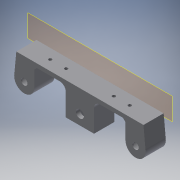
# Autodesk Inventor part: Bed Slide
Saved by Autodesk Inventor 2016 (Build 200138000, 138)
## iProperties
Created: 2016-04-23
Part Number: Bed Slide
Material: Generic
Document SubType Name: Modeling
Designer: Scott
Density: 1 g/cm^3
Appearance: Default
Author: Scott
Autodesk Inventor part; units mm, degrees
ref_plane "YZ Plane" through (0, 0, 0) normal (1, 0, 0) x (0, 1, 0)
ref_plane "XZ Plane" through (0, 0, 0) normal (0, 1, 0) x (-1, 0, 0)
ref_plane "XY Plane" through (0, 0, 0) normal (0, 0, 1) x (1, 0, 0)
ref_plane "Work Plane1" through (0, 0, -76.2) normal (0, 0, 1) x (1, 0, 0)
sketch "Sketch1" plane through (0, 0, -76.2) normal (0, 0, 1) x (1, 0, 0)
  line L0 (-80, -10.16) -> (80, -10.16) projected
  circle A0 centre (70, -38.1) radius 4 projected
  circle A1 centre (-70, -38.1) radius 4 projected
  arc A2 (82.7105, -38.1) -> (57.2895, -38.1) centre (70, -38.1) ccw projected
  arc A3 (57.2895, -38.1) -> (82.4735, -35.6569) centre (70, -38.1) ccw
  arc A4 (-82.4735, -35.6569) -> (-57.2895, -38.1) centre (-70, -38.1) ccw
  line L1 (82.7105, -38.1) -> (80, -10.16)
  line L2 (-82.7105, -38.1) -> (-80, -10.16)
  circle A5 centre (0, -38.1) radius 5.08
  line L3 (17.78, -25.4) -> (17.78, -50.8)
  line L4 (17.78, -50.8) -> (-17.78, -50.8)
  line L5 (-17.78, -50.8) -> (-17.78, -25.4)
  line L6 (-17.78, -25.4) -> (17.78, -50.8) construction
  line L7 (17.78, -25.4) -> (-17.78, -50.8) construction
  line L8 (80, -10.16) -> (-80, -10.16)
  line L9 (-17.78, -15.24) -> (-57.2895, -15.24)
  line L10 (17.78, -15.24) -> (57.2895, -15.24)
  line L11 (57.2895, -38.1) -> (57.2895, -15.24)
  line L12 (-57.2895, -38.1) -> (-57.2895, -15.24)
  line L13 (-17.78, -38.1) -> (-17.78, -15.24)
  line L14 (17.78, -38.1) -> (17.78, -15.24)
  point P0 (0, 0)
  dimension "d0" = 10.16
  dimension "d2" = 35.56
  dimension "d3" = 25.4
  constraints: 28 end point, 5 point on circle, 4 midpoint, 4 point on line, 3 centre point, 2 coincident, 2 horizontal, 2 perpendicular, 1 concentric, 1 parallel, 1 tangent
  measures "d0" diameter of A5
  measures "d2" distance of L3.end L4.end
  measures "d3" distance of L3.start L3.end
extrude "Extrusion1" add sketch "Sketch1" along normal blind 25.4 contours L0 L1 A2 L11 L10 L14 L3 L4 L5 L13 L9 L12 A4 L2 | L1 A3 A2 | A2 L1
sketch "Sketch2" plane through (0, 0, -76.2) normal (0, 0, -1) x (-1, 0, 0)
  circle A0 centre (-70, -38.1) radius 4 projected
  circle A1 centre (-70, -38.1) radius 7.5
  circle A2 centre (70, -38.1) radius 4 projected
  circle A3 centre (70, -38.1) radius 7.5
  point P0 (0, 0)
  dimension "d7" = 15
  dimension "d8" = 15
  constraints: 2 centre point, 2 coincident
  measures "d7" diameter of A1
  measures "d8" diameter of A3
extrude "Extrusion2" cut sketch "Sketch2" against normal blind 24
sketch "Sketch3" plane through (-17.78, -50.8, -76.2) normal (0, -1, 0) x (1, 0, 0)
  line L0 (0, 0) -> (35.56, 0) projected
  line L1 (0, 0) -> (0, 25.4) projected
  line L2 (0, 25.4) -> (35.56, 25.4) projected
  line L3 (35.56, 0) -> (35.56, 25.4) projected
  line L4 (12.7, 0) -> (12.7, 25.4) projected
  line L5 (22.86, 0) -> (22.86, 25.4) projected
  line L6 (12.7, 25.4) -> (22.86, 25.4) projected
  line L7 (17.78, 25.4) -> (17.78, 20.32)
  line L8 (22.86, 20.32) -> (12.7, 20.32)
  line L9 (12.7, 20.32) -> (12.7, 10.16)
  line L10 (12.7, 10.16) -> (22.86, 10.16)
  line L11 (22.86, 10.16) -> (22.86, 20.32)
  line L12 (17.78, 10.16) -> (28.575, 10.16)
  line L13 (28.575, 10.16) -> (6.985, 10.16)
  line L14 (28.575, 10.16) -> (6.985, 10.16)
  line L15 (6.985, 10.16) -> (6.985, 6.604)
  line L16 (6.985, 6.604) -> (28.575, 6.604)
  line L17 (28.575, 6.604) -> (28.575, 10.16)
  line L18 (12.7, 5.334) -> (22.86, 5.334)
  line L19 (22.86, 5.334) -> (22.86, 7.874)
  line L20 (22.86, 7.874) -> (12.7, 7.874)
  line L21 (12.7, 7.874) -> (12.7, 5.334)
  line L22 (12.7, 5.334) -> (22.86, 7.874) construction
  line L23 (22.86, 5.334) -> (12.7, 7.874) construction
  point P0 (17.78, 76.2)
  point P1 (17.78, 6.604)
  dimension "d11" = 5.08
  dimension "d12" = 10.16
  dimension "d13" = 10.16
  dimension "d14" = 10.795
  dimension "d15" = 21.59
  dimension "d16" = 21.59
  dimension "d17" = 3.556
  dimension "d18" = 10.16
  dimension "d19" = 2.54
  constraints: 34 end point, 6 parallel, 5 midpoint, 3 horizontal, 3 perpendicular, 3 point on line, 1 vertical
  measures "d11" distance of L7.start L7.end
  measures "d12" distance of L10.end L9.end
  measures "d13" distance of L9.end L8.end
  measures "d14" distance of L12.start L12.end
  measures "d15" distance of L12.end L13.end
  measures "d16" distance of L16.end L15.end
  measures "d17" distance of L15.end L14.end
  measures "d18" distance of L20.end L19.end
  measures "d19" distance of L19.end L18.end
extrude "Extrusion3" cut sketch "Sketch3" against normal blind 21.59 contours L4 L16 L5 L18 | L16 L15 L13 L4 | L4 L20 L5 L16 | L8 L5 L10 L4 | L5 L12 L17 L16 | L4 L10 L5 L20
fillet "Fillet1" radius 10.795 2 edges at (-10.795, -29.21, -67.818) (10.795, -29.21, -67.818)
sketch "Sketch4" plane through (17.78, -15.24, -76.2) normal (0, -1, 0) x (1, 0, 0)
  line L0 (0, 0) -> (39.5095, 0) projected
  line L1 (0, 25.4) -> (39.5095, 25.4) projected
  line L2 (-75.0695, 0) -> (-35.56, 0) projected
  line L3 (62.22, 25.4) -> (-97.78, 25.4) projected
  line L4 (-97.78, -170.15) -> (-97.78, 69.85) projected
  line L5 (62.22, -170.15) -> (-97.78, -170.15) projected
  line L6 (62.22, 69.85) -> (62.22, -170.15) projected
  line L7 (-97.78, 69.85) -> (62.22, 69.85) projected
  line L8 (62.22, 0) -> (62.22, 25.4) projected
  line L9 (62.22, 12.7) -> (32.22, 12.7)
  line L10 (32.22, 12.7) -> (12.22, 12.7)
  circle A0 centre (32.22, 12.7) radius 2
  circle A1 centre (12.22, 12.7) radius 2
  line L11 (62.22, 0) -> (-97.78, 0) projected
  line L12 (-17.78, 0) -> (-17.78, 2.4889)
  circle A2 centre (-67.78, 12.7) radius 2
  circle A3 centre (-47.78, 12.7) radius 2
  point P0 (-17.78, 76.2)
  dimension "d23" = 30
  dimension "d24" = 20
  dimension "d25" = 4
  dimension "d26" = 4
  constraints: 6 end point, 4 centre point, 2 coincident, 2 midpoint, 2 symmetric about line, 1 horizontal, 1 point on line, 1 vertical, 2 other
  measures "d23" distance of L9.start L9.end
  measures "d24" distance of L9.end L10.end
  measures "d25" diameter of A0
  measures "d26" diameter of A1
extrude "Extrusion4" cut sketch "Sketch4" against normal blind 25.4 contours A0 L10 L9 | L9 L10 A0 | A1 | A2 | A3
chamfer "Chamfer1" distance 3.175 angle 45 2 edges at (57.2895, -15.24, -63.5) (-57.2895, -15.24, -63.5)
fillet "Fillet2" radius 7.62 2 edges at (17.78, -15.24, -63.5) (-17.78, -15.24, -63.5)
body "Solid1"
